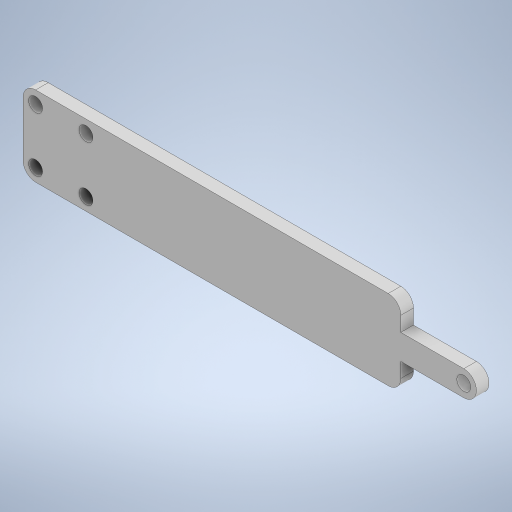
# Autodesk Inventor part: Arm2
Saved by Autodesk Inventor 2023 (Build 270158000, 158)
## iProperties
Created: 2023-12-17
Part Number: Arm2
Material: Generic
Document SubType Name: Modeling
Designer: Mustapha
Density: 1 g/cm^3
Appearance: Default
Author: Mustapha
Autodesk Inventor part; units mm, degrees
ref_plane "YZ Plane" through (0, 0, 0) normal (1, 0, 0) x (0, 1, 0)
ref_plane "XZ Plane" through (0, 0, 0) normal (0, 1, 0) x (-1, 0, 0)
ref_plane "XY Plane" through (0, 0, 0) normal (0, 0, 1) x (1, 0, 0)
sketch "Sketch1" plane through (0, 0, 0) normal (0, 0, 1) x (1, 0, 0)
  line L0 (5, 0) -> (145, 0)
  line L1 (150, 5) -> (150, 26.714)
  line L2 (145, 31.714) -> (5, 31.714)
  line L3 (0, 26.714) -> (0, 5)
  arc A0 (5, 31.714) -> (0, 26.714) centre (5, 26.714) ccw
  arc A1 (0, 5) -> (5, 0) centre (5, 5) ccw
  circle A2 centre (5, 5) radius 2.75
  circle A3 centre (5, 26.714) radius 2.75
  circle A4 centre (25, 26.714) radius 2.75
  circle A5 centre (25, 5) radius 2.75
  arc A6 (150, 26.714) -> (145, 31.714) centre (145, 26.714) ccw
  arc A7 (145, 0) -> (150, 5) centre (145, 5) ccw
  line L4 (175, 20.857) -> (120, 20.857)
  line L5 (120, 20.857) -> (120, 10.857)
  line L6 (120, 10.857) -> (175, 10.857)
  line L7 (180, 15.857) -> (180, 15.857)
  line L8 (180, 20.857) -> (120, 10.857) construction
  line L9 (120, 20.857) -> (180, 10.857) construction
  circle A8 centre (175, 15.857) radius 2.75
  arc A9 (180, 15.857) -> (175, 20.857) centre (175, 15.857) ccw
  arc A10 (175, 10.857) -> (180, 15.857) centre (175, 15.857) ccw
  point P0 (0, 0)
  point P1 (150, 31.714)
  point P2 (150, 0)
  point P3 (150, 15.857)
  point P4 (0, 15.857)
  point P5 (180, 15.857)
  point P6 (150, 10.857)
  point P7 (150, 20.857)
  dimension "d0" = 150
  dimension "d1" = 31.714
  dimension "d2" = 5
  dimension "d3" = 5.5
  dimension "d4" = 5.5
  dimension "d5" = 21.714
  dimension "d8" = 20
  dimension "d13" = 5
  dimension "d14" = 10
  dimension "d15" = 60
  dimension "d16" = 5.5
  dimension "d17" = 5
  dimension "d18" = 5
  constraints: 20 end point, 12 point on circle, 12 tangent, 11 centre point, 10 point on line, 5 midpoint, 4 parallel, 3 equal radius, 3 horizontal, 2 coincident, 2 perpendicular, 4 other
  measures "d0" distance of point (150, 15.857) point (0, 15.857)
  measures "d1" distance of point (150, 0) point (150, 31.714)
  measures "d2" radius of A0
  measures "d3" diameter of A3
  measures "d4" diameter of A2
  measures "d5" distance of A1.centre A0.centre
  measures "d8" distance of A3.centre A4.centre
  measures "d13" radius of A6
  measures "d14" distance between parallel lines of L6 L4
  measures "d15" horizontal distance of point (180, 15.857) L5.end
  measures "d16" diameter of A8
  measures "d17" distance from line of L7 A8.centre
  measures "d18" radius of A9
extrude "Extrusion1" add sketch "Sketch1" along normal blind 5
body "Solid1"
